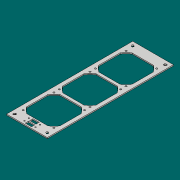
# Autodesk Inventor part: top_panel_2
Saved by Autodesk Inventor 2018.2 (Build 222227000, 227)
## iProperties
Created: 2019-10-14
Part Number: top_panel_2
Material: アルミニウム 6061
Document SubType Name: Modeling
Designer: gisen
Density: 2.7 g/cm^3
Appearance: アルミニウム - フラット
Author: gisen
Autodesk Inventor part; units mm, degrees
ref_plane "YZ Plane" through (0, 0, 0) normal (1, 0, 0) x (0, 1, 0)
ref_plane "XZ Plane" through (0, 0, 0) normal (0, 1, 0) x (-1, 0, 0)
ref_plane "XY Plane" through (0, 0, 0) normal (0, 0, 1) x (1, 0, 0)
sketch "スケッチ1" plane through (0, 0, 0) normal (0, 0, 1) x (1, 0, 0)
  line L0 (-55, -170) -> (55, -170)
  line L1 (55, -170) -> (55, 170)
  line L2 (55, 170) -> (-55, 170)
  line L3 (-55, 170) -> (-55, -170)
  line L4 (-55, -170) -> (55, 170) construction
  line L5 (55, -170) -> (-55, 170) construction
  line L6 (-55, 140) -> (-50, 140) construction
  line L7 (-50, 140) -> (-25, 165) construction
  line L8 (-25, 165) -> (-25, 170) construction
  line L9 (-46, 51) -> (46, 51) construction
  line L10 (46, 51) -> (46, 143) construction
  line L11 (46, 143) -> (-46, 143) construction
  line L12 (-46, 143) -> (-46, 51) construction
  line L13 (-46, 51) -> (46, 143) construction
  line L14 (46, 51) -> (-46, 143) construction
  line L15 (-46, 2.5) -> (46, 2.5) construction
  line L16 (46, 2.5) -> (46, 46) construction
  line L17 (46, 46) -> (-46, 46) construction
  line L18 (-46, 46) -> (-46, 2.5) construction
  line L19 (-46, 2.5) -> (46, 46) construction
  line L20 (46, 2.5) -> (-46, 46) construction
  line L21 (0, 0) -> (0, 97) construction
  circle A0 centre (0, 97) radius 53 construction
  line L22 (-44.7, 52.3) -> (44.7, 52.3) construction
  line L23 (44.7, 52.3) -> (44.7, 141.7) construction
  line L24 (44.7, 141.7) -> (-44.7, 141.7) construction
  line L25 (-44.7, 141.7) -> (-44.7, 52.3) construction
  line L26 (-44.7, 52.3) -> (44.7, 141.7) construction
  line L27 (44.7, 52.3) -> (-44.7, 141.7) construction
  arc A1 (-28.4765, 141.7) -> (-44.7, 125.4765) centre (0, 97) ccw
  arc A2 (-44.7, 68.5235) -> (-28.4765, 52.3) centre (0, 97) ccw
  arc A3 (28.4765, 52.3) -> (44.7, 68.5235) centre (0, 97) ccw
  arc A4 (44.7, 125.4765) -> (28.4765, 141.7) centre (0, 97) ccw
  line L28 (-28.4765, 141.7) -> (28.4765, 141.7)
  line L29 (-44.7, 125.4765) -> (-44.7, 68.5235)
  line L30 (-28.4765, 52.3) -> (28.4765, 52.3)
  line L31 (44.7, 68.5235) -> (44.7, 125.4765)
  line L32 (-41.25, 55.75) -> (41.25, 55.75) construction
  line L33 (41.25, 55.75) -> (41.25, 138.25) construction
  line L34 (41.25, 138.25) -> (-41.25, 138.25) construction
  line L35 (-41.25, 138.25) -> (-41.25, 55.75) construction
  line L36 (-41.25, 55.75) -> (41.25, 138.25) construction
  line L37 (41.25, 55.75) -> (-41.25, 138.25) construction
  circle A5 centre (-41.25, 138.25) radius 2.25
  circle A6 centre (-41.25, 55.75) radius 2.25
  circle A7 centre (41.25, 55.75) radius 2.25
  circle A8 centre (41.25, 138.25) radius 2.25
  circle A9 centre (-45, 160) radius 2.25
  circle A10 centre (45, 160) radius 2.25
  circle A11 centre (45, -160) radius 2.25
  circle A12 centre (-45, -160) radius 2.25
  line L38 (-55, 0) -> (55, 0) construction
  circle A13 centre (-41.25, -41.25) radius 2.25
  arc A14 (-44.7, -28.4765) -> (-28.4765, -44.7) centre (0, 0) ccw
  line L39 (-28.4765, -44.7) -> (28.4765, -44.7)
  arc A15 (28.4765, -44.7) -> (44.7, -28.4765) centre (0, 0) ccw
  circle A16 centre (41.25, -41.25) radius 2.25
  line L40 (44.7, -28.4765) -> (44.7, 28.4765)
  circle A17 centre (41.25, 41.25) radius 2.25
  arc A18 (44.7, 28.4765) -> (28.4765, 44.7) centre (0, 0) ccw
  line L41 (-28.4765, 44.7) -> (28.4765, 44.7)
  circle A19 centre (-41.25, 41.25) radius 2.25
  arc A20 (-28.4765, 44.7) -> (-44.7, 28.4765) centre (0, 0) ccw
  line L42 (-44.7, 28.4765) -> (-44.7, -28.4765)
  circle A21 centre (-41.25, -138.25) radius 2.25
  arc A22 (-44.7, -125.4765) -> (-28.4765, -141.7) centre (0, -97) ccw
  line L43 (-28.4765, -141.7) -> (28.4765, -141.7)
  arc A23 (28.4765, -141.7) -> (44.7, -125.4765) centre (0, -97) ccw
  circle A24 centre (41.25, -138.25) radius 2.25
  line L44 (44.7, -125.4765) -> (44.7, -68.5235)
  circle A25 centre (41.25, -55.75) radius 2.25
  arc A26 (44.7, -68.5235) -> (28.4765, -52.3) centre (0, -97) ccw
  line L45 (-28.4765, -52.3) -> (28.4765, -52.3)
  circle A27 centre (-41.25, -55.75) radius 2.25
  arc A28 (-28.4765, -52.3) -> (-44.7, -68.5235) centre (0, -97) ccw
  line L46 (-44.7, -68.5235) -> (-44.7, -125.4765)
  point P0 (0, 24.25)
  point P1 (0, 24.25)
  dimension "d12" = 106
  dimension "d0" = 110
  dimension "d1" = 340
  dimension "d2" = 135
  dimension "d3" = 30
  dimension "d4" = 30
  dimension "d5" = 5
  dimension "d6" = 92
  dimension "d7" = 92
  dimension "d8" = 92
  dimension "d9" = 43.5
  dimension "d10" = 5
  dimension "d11" = 2.5
  dimension "d13" = 89.4
  dimension "d14" = 89.4
  dimension "d15" = 82.5
  dimension "d16" = 82.5
  dimension "d17" = 4.5
  dimension "d25" = 4.5
  dimension "d26" = 10
  dimension "d27" = 10
  dimension "d28" = 10
  dimension "d29" = 10
  dimension "d30" = 10
  dimension "d31" = 10
  dimension "d32" = 10
  dimension "d33" = 10
  dimension "d45" = 97
  dimension "d80" = 0
  constraints: 94 end point, 28 centre point, 24 point on circle, 15 coincident, 13 midpoint, 11 point on line, 10 parallel, 8 perpendicular, 6 equal radius, 6 horizontal, 2 vertical, 1 collinear, 66 other
  measures "d0" distance of L2.end L1.end
  measures "d1" distance of L1.end L0.end
  measures "d2" angle of L7 L6
  measures "d3" distance between parallel lines of L8 L3
  measures "d4" distance between parallel lines of L2 L6
  measures "d5" distance of L7.end L8.end
  measures "d6" distance of L11.end L10.end
  measures "d7" distance of L10.end L9.end
  measures "d8" distance of L17.end L16.end
  measures "d9" distance of L16.end L15.end
  measures "d10" distance between parallel lines of L17 L9
  measures "d11" distance from line of L21.start L15
  measures "d13" distance of L24.end L23.end
  measures "d14" distance of L23.end L22.end
  measures "d15" distance of L34.end L33.end
  measures "d16" distance of L33.end L32.end
  measures "d17" diameter of A5
  measures "d25" diameter of A9
  measures "d26" distance from line of A9.centre L2
  measures "d27" distance from line of L3 A9.centre
  measures "d28" distance from line of L2 A10.centre
  measures "d29" distance from line of L1 A10.centre
  measures "d30" distance from line of L1 A11.centre
  measures "d31" distance from line of L0 A11.centre
  measures "d32" distance from line of L0 A12.centre
  measures "d33" distance from line of L3 A12.centre
  measures "d45" distance of A6.centre A13.centre
  measures "d80" distance of L21.start A14.centre
extrude "押し出し1" add sketch "スケッチ1" along normal blind 3
sketch "スケッチ2" plane through (0, 0, 3) normal (0, 0, 1) x (1, 0, 0)
  circle A0 centre (-45, 160) radius 2.25 construction
  circle A1 centre (45, -160) radius 2.25 construction
  circle A2 centre (-45, -160) radius 2.25 construction
  circle A3 centre (-43, 158) radius 2.75 construction
  line L0 (55, 170) -> (-55, 170) projected
  line L1 (-55, 170) -> (-55, -170) projected
  line L2 (-43.7153, 161.8472) -> (-41.4298, 160.2577)
  line L3 (-45.2577, 156.4298) -> (-46.8472, 158.7153)
  circle A4 centre (-45, 160) radius 2.25 construction
  arc A5 (-43.7153, 161.8472) -> (-46.8472, 158.7153) centre (-45, 160) ccw
  arc A6 (-45.2577, 156.4298) -> (-41.4298, 160.2577) centre (-43, 158) ccw
  line L4 (55, 170) -> (-55, 170) construction
  line L5 (0, 170) -> (0, -170) construction
  line L6 (-55, -170) -> (55, -170) construction
  line L7 (-55, 0) -> (55, 0) construction
  line L8 (55, -170) -> (55, 170) construction
  circle A7 centre (45, 160) radius 2.25 construction
  circle A8 centre (43, 158) radius 2.75 construction
  line L9 (43.7153, 161.8472) -> (41.4298, 160.2577)
  line L10 (45.2577, 156.4298) -> (46.8472, 158.7153)
  circle A9 centre (45, 160) radius 2.25 construction
  arc A10 (46.8472, 158.7153) -> (43.7153, 161.8472) centre (45, 160) ccw
  arc A11 (41.4298, 160.2577) -> (45.2577, 156.4298) centre (43, 158) ccw
  circle A12 centre (-45, -160) radius 2.25 construction
  circle A13 centre (-43, -158) radius 2.75 construction
  line L11 (-43.7153, -161.8472) -> (-41.4298, -160.2577)
  line L12 (-45.2577, -156.4298) -> (-46.8472, -158.7153)
  circle A14 centre (-45, -160) radius 2.25 construction
  arc A15 (-46.8472, -158.7153) -> (-43.7153, -161.8472) centre (-45, -160) ccw
  arc A16 (-41.4298, -160.2577) -> (-45.2577, -156.4298) centre (-43, -158) ccw
  circle A17 centre (45, -160) radius 2.25 construction
  line L13 (45.2577, -156.4298) -> (46.8472, -158.7153)
  arc A18 (45.2577, -156.4298) -> (41.4298, -160.2577) centre (43, -158) ccw
  circle A19 centre (43, -158) radius 2.75 construction
  line L14 (43.7153, -161.8472) -> (41.4298, -160.2577)
  circle A20 centre (45, -160) radius 2.25 construction
  arc A21 (43.7153, -161.8472) -> (46.8472, -158.7153) centre (45, -160) ccw
  point P0 (0, 0)
  dimension "d38" = 5.5
  dimension "d39" = 12
  dimension "d40" = 12
  constraints: 28 point on circle, 27 symmetric about line, 20 end point, 15 centre point, 8 coincident, 4 midpoint, 2 horizontal, 2 tangent, 1 vertical, 25 other
  measures "d38" diameter of A3
  measures "d39" distance from line of A3.centre L0
  measures "d40" distance from line of L1 A3.centre
extrude "押し出し2" cut sketch "スケッチ2" against normal through all
sketch "スケッチ3" plane through (0, 0, 3) normal (0, 0, 1) x (1, 0, 0)
  line L0 (-55, -170) -> (55, -170) construction
  line L1 (-55, 170) -> (-55, -170) construction
  line L2 (55, -170) -> (55, 170) construction
  line L3 (0, -170) -> (0, -116.79) construction
  arc A0 (-17.4739, -147.55) -> (-17.4739, -162.45) centre (-15, -155) ccw construction
  line L4 (-17.4739, -147.55) -> (-12.5261, -147.55) construction
  line L5 (-12.5261, -162.45) -> (-17.4739, -162.45) construction
  arc A1 (-12.5261, -147.55) -> (-17.4739, -147.55) centre (-15, -155) ccw construction
  arc A2 (-12.5261, -162.45) -> (-12.5261, -147.55) centre (-15, -155) ccw construction
  arc A3 (-17.4739, -162.45) -> (-12.5261, -162.45) centre (-15, -155) ccw construction
  line L6 (-17.4755, -162.46) -> (-12.5245, -162.46)
  arc A4 (-12.5245, -162.46) -> (-12.5245, -147.54) centre (-15, -155) ccw
  line L7 (-12.5245, -147.54) -> (-17.4755, -147.54)
  arc A5 (-17.4755, -147.54) -> (-17.4755, -162.46) centre (-15, -155) ccw
  line L8 (17.4755, -162.46) -> (12.5245, -162.46)
  arc A6 (12.5245, -147.54) -> (12.5245, -162.46) centre (15, -155) ccw
  line L9 (12.5245, -147.54) -> (17.4755, -147.54)
  arc A7 (17.4755, -162.46) -> (17.4755, -147.54) centre (15, -155) ccw
  point P0 (0, 0)
  dimension "d50" = 15.7
  dimension "d51" = 14.9
  dimension "d52" = 15
  dimension "d53" = 15
  dimension "d54" = 40
  dimension "d55" = 0.01
  constraints: 17 point on circle, 14 end point, 8 centre point, 5 symmetric about line, 3 parallel, 1 horizontal, 1 midpoint, 1 vertical, 5 other
  measures "d50" diameter of A0
  measures "d51" distance between parallel lines of L5 L4
  measures "d52" distance from line of L0 A0.centre
  measures "d53" distance from line of L3 A0.centre
  measures "d54" distance from line of A0.centre L1
  measures "d55" radial gap between concentric circles of A0 A5
extrude "押し出し3" [suppressed]
sketch "スケッチ4" plane through (0, 0, 3) normal (0, 0, 1) x (1, 0, 0)
  line L0 (-55, 170) -> (-55, -170) projected
  line L1 (-55, 170) -> (55, 170)
  line L2 (55, 170) -> (55, 167)
  line L3 (55, 167) -> (-55, 167)
  line L4 (-55, 167) -> (-55, 170)
  point P0 (0, 0)
  dimension "d58" = 3
  constraints: 8 end point, 2 parallel, 1 horizontal, 1 perpendicular
  measures "d58" distance between parallel lines of L3 L1
extrude "押し出し4" [suppressed]
sketch "スケッチ6" plane through (0, 0, 3) normal (0, 0, 1) x (1, 0, 0)
  line L0 (-55, 170) -> (-55, -170) construction
  line L1 (-55, -170) -> (-25, -170) construction
  line L2 (-25, -170) -> (-25, -140) construction
  line L3 (-25, -140) -> (-55, -140) construction
  line L4 (-55, -140) -> (-55, -170) construction
  line L5 (-40, -100) -> (-40, -140) construction
  line L6 (-46.25, -120) -> (-46.25, -105) construction
  line L7 (-46.25, -120) -> (-46.25, -135) construction
  line L8 (-33.75, -120) -> (-33.75, -105) construction
  line L9 (-33.75, -120) -> (-33.75, -135) construction
  circle A0 centre (-46.25, -105) radius 1.65
  circle A1 centre (-33.75, -105) radius 1.65 construction
  circle A2 centre (-33.75, -135) radius 1.65 construction
  circle A3 centre (-46.25, -135) radius 1.65
  line L10 (-50.75, -128.5) -> (-41.75, -128.5)
  line L11 (-41.75, -128.5) -> (-41.75, -111.5)
  line L12 (-41.75, -111.5) -> (-50.75, -111.5)
  line L13 (-50.75, -111.5) -> (-50.75, -128.5)
  line L14 (-50.75, -128.5) -> (-41.75, -111.5) construction
  line L15 (-41.75, -128.5) -> (-50.75, -111.5) construction
  line L16 (-38.25, -128.5) -> (-29.25, -128.5) construction
  line L17 (-29.25, -128.5) -> (-29.25, -111.5) construction
  line L18 (-29.25, -111.5) -> (-38.25, -111.5) construction
  line L19 (-38.25, -111.5) -> (-38.25, -128.5) construction
  line L20 (-38.25, -128.5) -> (-29.25, -111.5) construction
  line L21 (-29.25, -128.5) -> (-38.25, -111.5) construction
  line L22 (-52.5, -100) -> (-27.5, -100) construction
  line L23 (-46.25, -120) -> (-40, -120) construction
  line L24 (-33.75, -120) -> (-40, -120) construction
  circle A4 centre (-46.25, -95) radius 1.65
  circle A5 centre (-46.25, -65) radius 1.65
  line L25 (-50.75, -71.5) -> (-41.75, -71.5)
  line L26 (-41.75, -71.5) -> (-41.75, -88.5)
  line L27 (-41.75, -88.5) -> (-50.75, -88.5)
  line L28 (-50.75, -88.5) -> (-50.75, -71.5)
  point P0 (0, 0)
  point P1 (-36.875, -120)
  point P2 (-43.125, -120)
  dimension "d64" = 30
  dimension "d65" = 30
  dimension "d68" = 30
  dimension "d69" = 3.3
  dimension "d70" = 9
  dimension "d71" = 17
  dimension "d75" = 25
  dimension "d77" = 6.25
  dimension "d78" = 40
  dimension "d79" = 15
  constraints: 56 end point, 13 equal length, 11 midpoint, 6 centre point, 6 symmetric about line, 5 vertical, 4 coincident, 4 horizontal, 3 equal radius, 3 perpendicular, 1 horizontal alignment, 2 other
  measures "d64" distance of L3.end L2.end
  measures "d65" distance of L2.end L1.end
  measures "d68" distance of L7.end L6.end
  measures "d69" diameter of A0
  measures "d70" distance of L12.end L11.end
  measures "d71" distance of L11.end L10.end
  measures "d75" distance of L22.start L22.end
  measures "d77" distance of L6.start L23.end
  measures "d78" distance between parallel lines of L3 L22
  measures "d79" distance between parallel lines of L0 L5
extrude "押し出し6" [suppressed]
sketch "スケッチ8" plane through (0, 0, 3) normal (0, 0, 1) x (1, 0, 0)
  line L0 (-55, -170) -> (55, -170) construction
  line L1 (-55, -170) -> (55, -170) construction
  line L2 (0, -170) -> (0, -141.7) construction
  line L3 (-28.4765, -141.7) -> (28.4765, -141.7) construction
  line L4 (-55, 170) -> (-55, -170) construction
  line L5 (-55, -140) -> (-50, -140) construction
  line L6 (-50, -140) -> (-25, -165) construction
  line L7 (-25, -165) -> (-25, -170) construction
  line L8 (-20, -161.5) -> (20, -161.5) construction
  line L9 (-20, -149.5) -> (20, -149.5) construction
  line L10 (-8.5, -154) -> (8.5, -154)
  line L11 (8.5, -154) -> (8.5, -145)
  line L12 (8.5, -145) -> (-8.5, -145)
  line L13 (-8.5, -145) -> (-8.5, -154)
  line L14 (-8.5, -154) -> (8.5, -145) construction
  line L15 (8.5, -154) -> (-8.5, -145) construction
  line L16 (-8.5, -166) -> (8.5, -166)
  line L17 (8.5, -166) -> (8.5, -157)
  line L18 (8.5, -157) -> (-8.5, -157)
  line L19 (-8.5, -157) -> (-8.5, -166)
  line L20 (-8.5, -166) -> (8.5, -157) construction
  line L21 (8.5, -166) -> (-8.5, -157) construction
  circle A0 centre (-15, -149.5) radius 1.65
  line L22 (-15, -149.5) -> (-15, -161.5) construction
  circle A1 centre (-15, -161.5) radius 1.65
  circle A2 centre (15, -149.5) radius 1.65
  circle A3 centre (15, -161.5) radius 1.65
  point P0 (0, 0)
  point P1 (0, -161.5)
  point P2 (0, -149.5)
  dimension "d84" = 5
  dimension "d85" = 135
  dimension "d86" = 5
  dimension "d87" = 30
  dimension "d88" = 40
  dimension "d89" = 12
  dimension "d90" = 8.5
  dimension "d91" = 7.8
  dimension "d92" = 17
  dimension "d93" = 9
  dimension "d94" = 3.3
  dimension "d95" = 15
  constraints: 38 end point, 8 midpoint, 6 point on line, 5 perpendicular, 4 centre point, 4 horizontal, 4 parallel, 3 equal length, 2 symmetric about line, 1 coincident, 1 equal radius, 2 other
  measures "d84" distance of L5.start L5.end
  measures "d85" angle of L5 L6
  measures "d86" distance of L6.end L7.end
  measures "d87" distance from line of L7 L0.start
  measures "d88" distance of L8.start L8.end
  measures "d89" distance of point (0, -161.5) point (0, -149.5)
  measures "d90" distance from line of L0 point (0, -161.5)
  measures "d91" distance of point (0, -149.5) L2.end
  measures "d92" distance of L12.end L11.end
  measures "d93" distance of L11.end L10.end
  measures "d94" diameter of A0
  measures "d95" distance from line of L2 L22.start
extrude "押し出し7" cut sketch "スケッチ8" against normal through all
sketch "スケッチ5" plane through (0, 0, 3) normal (0, 0, 1) x (1, 0, 0)
  line L0 (-55, -170) -> (55, -170) construction
  line L1 (55, -170) -> (55, 170) construction
  line L2 (55, 170) -> (-55, 170) construction
  line L3 (-55, 170) -> (-55, -170) construction
  circle A0 centre (-41.25, 138.25) radius 2.25 construction
  circle A1 centre (-41.25, 55.75) radius 2.25 construction
  circle A2 centre (41.25, 55.75) radius 2.25 construction
  circle A3 centre (41.25, 138.25) radius 2.25 construction
  line L4 (43.7153, -161.8472) -> (41.4298, -160.2577) construction
  arc A4 (45.2577, -156.4298) -> (41.4298, -160.2577) centre (43, -158) ccw construction
  line L5 (45.2577, -156.4298) -> (46.8472, -158.7153) construction
  arc A5 (43.7153, -161.8472) -> (46.8472, -158.7153) centre (45, -160) ccw construction
  circle A6 centre (-41.25, -41.25) radius 2.25 construction
  circle A7 centre (41.25, -41.25) radius 2.25 construction
  circle A8 centre (41.25, 41.25) radius 2.25 construction
  circle A9 centre (-41.25, 41.25) radius 2.25 construction
  line L6 (-28.4765, 141.7) -> (28.4765, 141.7) construction
  arc A10 (44.7, 125.4765) -> (28.4765, 141.7) centre (0, 97) ccw construction
  line L7 (44.7, 125.4765) -> (44.7, 68.5235) construction
  arc A11 (28.4765, 52.3) -> (44.7, 68.5235) centre (0, 97) ccw construction
  line L8 (28.4765, 52.3) -> (-28.4765, 52.3) construction
  arc A12 (-44.7, 68.5235) -> (-28.4765, 52.3) centre (0, 97) ccw construction
  line L9 (-44.7, 68.5235) -> (-44.7, 125.4765) construction
  arc A13 (-28.4765, 141.7) -> (-44.7, 125.4765) centre (0, 97) ccw construction
  line L10 (-44.7, -28.4765) -> (-44.7, 28.4765) construction
  arc A14 (-28.4765, 44.7) -> (-44.7, 28.4765) centre (0, 0) ccw construction
  line L11 (-28.4765, 44.7) -> (28.4765, 44.7) construction
  arc A15 (44.7, 28.4765) -> (28.4765, 44.7) centre (0, 0) ccw construction
  line L12 (44.7, 28.4765) -> (44.7, -28.4765) construction
  arc A16 (28.4765, -44.7) -> (44.7, -28.4765) centre (0, 0) ccw construction
  line L13 (28.4765, -44.7) -> (-28.4765, -44.7) construction
  arc A17 (-44.7, -28.4765) -> (-28.4765, -44.7) centre (0, 0) ccw construction
  line L14 (41.4298, 160.2577) -> (43.7153, 161.8472) construction
  arc A18 (46.8472, 158.7153) -> (43.7153, 161.8472) centre (45, 160) ccw construction
  line L15 (46.8472, 158.7153) -> (45.2577, 156.4298) construction
  arc A19 (41.4298, 160.2577) -> (45.2577, 156.4298) centre (43, 158) ccw construction
  line L16 (-45.2577, 156.4298) -> (-46.8472, 158.7153) construction
  arc A20 (-43.7153, 161.8472) -> (-46.8472, 158.7153) centre (-45, 160) ccw construction
  line L17 (-43.7153, 161.8472) -> (-41.4298, 160.2577) construction
  arc A21 (-45.2577, 156.4298) -> (-41.4298, 160.2577) centre (-43, 158) ccw construction
  line L18 (-41.4298, -160.2577) -> (-43.7153, -161.8472) construction
  arc A22 (-46.8472, -158.7153) -> (-43.7153, -161.8472) centre (-45, -160) ccw construction
  line L19 (-46.8472, -158.7153) -> (-45.2577, -156.4298) construction
  arc A23 (-41.4298, -160.2577) -> (-45.2577, -156.4298) centre (-43, -158) ccw construction
  line L20 (-54.7, 169.7) -> (54.7, 169.7)
  line L21 (54.7, 169.7) -> (54.7, -169.7)
  line L22 (54.7, -169.7) -> (-54.7, -169.7)
  line L23 (-54.7, -169.7) -> (-54.7, 169.7)
  line L24 (-44.7, -125.4765) -> (-44.7, -68.5235) projected
  arc A24 (-28.4765, -52.3) -> (-44.7, -68.5235) centre (0, -97) ccw projected
  line L25 (-28.4765, -52.3) -> (28.4765, -52.3) projected
  arc A25 (44.7, -68.5235) -> (28.4765, -52.3) centre (0, -97) ccw projected
  line L26 (44.7, -68.5235) -> (44.7, -125.4765) projected
  arc A26 (28.4765, -141.7) -> (44.7, -125.4765) centre (0, -97) ccw projected
  line L27 (28.4765, -141.7) -> (-28.4765, -141.7) projected
  arc A27 (-44.7, -125.4765) -> (-28.4765, -141.7) centre (0, -97) ccw projected
  dimension "d61" = 0.3
  constraints: 8 end point, 3 other
  measures "d61" distance between parallel lines of L2 L20
extrude "押し出し5" cut sketch "スケッチ5" against normal through all contours L20 L21 L22 L23 | L24 A24 L25 A25 L26 A26 L27 A27 keep common part
equation "\"d4\" = d3"
equation "\"d11\" = 0.5 * d10"
equation "\"d27\" = d26"
equation "\"d28\" = d26"
equation "\"d29\" = d26"
equation "\"d30\" = d26"
equation "\"d31\" = d26"
equation "\"d32\" = d26"
equation "\"d33\" = d26"
equation "\"d45\" = d7 + d10"
equation "\"d77\" = 0.25 * d75"
